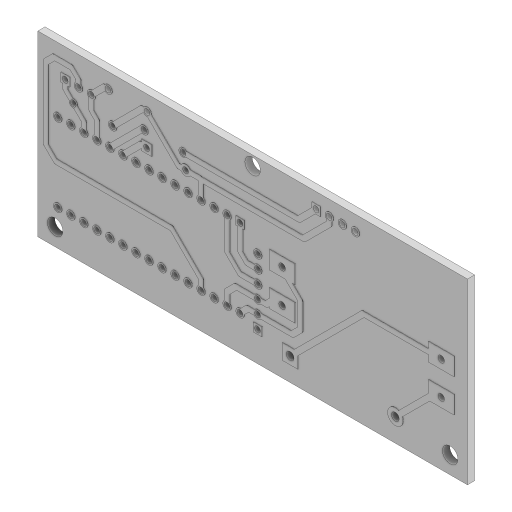
# Autodesk Inventor part: Деталь1
Saved by Autodesk Inventor 2024 (Build 280153020, 153B)
## iProperties
Created: 2023-07-24
Part Number: Деталь1
Material: Типовые
Document SubType Name: Modeling
Designer: Admin
Density: 1 g/cm^3
Appearance: По умолчанию
Author: Admin
Autodesk Inventor part; units mm, degrees
(part 1 of 3)
ref_plane "YZ Plane" through (0, 0, 0) normal (1, 0, 0) x (0, 1, 0)
ref_plane "XZ Plane" through (0, 0, 0) normal (0, 1, 0) x (-1, 0, 0)
ref_plane "XY Plane" through (0, 0, 0) normal (0, 0, 1) x (1, 0, 0)
sketch "Эскиз1" plane through (0, 0, 0) normal (0, 0, 1) x (1, 0, 0)
  line L0 (80.7425, 5.0309) -> (80.979, 4.9741)
  line L1 (80.979, 4.9741) -> (81.2037, 4.8811)
  line L2 (81.2037, 4.8811) -> (81.4111, 4.754)
  line L3 (81.4111, 4.754) -> (81.596, 4.596)
  line L4 (81.596, 4.596) -> (81.754, 4.4111)
  line L5 (81.754, 4.4111) -> (81.8811, 4.2037)
  line L6 (81.8811, 4.2037) -> (81.9741, 3.979)
  line L7 (81.9741, 3.979) -> (82.0309, 3.7425)
  line L8 (82.0309, 3.7425) -> (82.05, 3.5)
  line L9 (82.05, 3.5) -> (82.0309, 3.2575)
  line L10 (82.0309, 3.2575) -> (81.9741, 3.021)
  line L11 (81.9741, 3.021) -> (81.8811, 2.7963)
  line L12 (81.8811, 2.7963) -> (81.754, 2.5889)
  line L13 (81.754, 2.5889) -> (81.596, 2.404)
  line L14 (81.596, 2.404) -> (81.4111, 2.246)
  line L15 (81.4111, 2.246) -> (81.2037, 2.1189)
  line L16 (81.2037, 2.1189) -> (80.979, 2.0259)
  line L17 (80.979, 2.0259) -> (80.7425, 1.9691)
  line L18 (80.7425, 1.9691) -> (80.5, 1.95)
  line L19 (80.5, 1.95) -> (80.2575, 1.9691)
  line L20 (80.2575, 1.9691) -> (80.021, 2.0259)
  line L21 (80.021, 2.0259) -> (79.7963, 2.1189)
  line L22 (79.7963, 2.1189) -> (79.5889, 2.246)
  line L23 (79.5889, 2.246) -> (79.404, 2.404)
  line L24 (79.404, 2.404) -> (79.246, 2.5889)
  line L25 (79.246, 2.5889) -> (79.1189, 2.7963)
  line L26 (79.1189, 2.7963) -> (79.0259, 3.021)
  line L27 (79.0259, 3.021) -> (78.9691, 3.2575)
  line L28 (78.9691, 3.2575) -> (78.95, 3.5)
  line L29 (78.95, 3.5) -> (78.9691, 3.7425)
  line L30 (78.9691, 3.7425) -> (79.0259, 3.979)
  line L31 (79.0259, 3.979) -> (79.1189, 4.2037)
  line L32 (79.1189, 4.2037) -> (79.246, 4.4111)
  line L33 (79.246, 4.4111) -> (79.404, 4.596)
  line L34 (79.404, 4.596) -> (79.5889, 4.754)
  line L35 (79.5889, 4.754) -> (79.7963, 4.8811)
  line L36 (79.7963, 4.8811) -> (80.021, 4.9741)
  line L37 (80.021, 4.9741) -> (80.2575, 5.0309)
  line L38 (80.2575, 5.0309) -> (80.5, 5.05)
  line L39 (80.5, 5.05) -> (80.7425, 5.0309)
  line L40 (3.7425, 5.0309) -> (3.979, 4.9741)
  line L41 (3.979, 4.9741) -> (4.2037, 4.8811)
  line L42 (4.2037, 4.8811) -> (4.4111, 4.754)
  line L43 (4.4111, 4.754) -> (4.596, 4.596)
  line L44 (4.596, 4.596) -> (4.754, 4.4111)
  line L45 (4.754, 4.4111) -> (4.8811, 4.2037)
  line L46 (4.8811, 4.2037) -> (4.9741, 3.979)
  line L47 (4.9741, 3.979) -> (5.0309, 3.7425)
  line L48 (5.0309, 3.7425) -> (5.05, 3.5)
  line L49 (5.05, 3.5) -> (5.0309, 3.2575)
  line L50 (5.0309, 3.2575) -> (4.9741, 3.021)
  line L51 (4.9741, 3.021) -> (4.8811, 2.7963)
  line L52 (4.8811, 2.7963) -> (4.754, 2.5889)
  line L53 (4.754, 2.5889) -> (4.596, 2.404)
  line L54 (4.596, 2.404) -> (4.4111, 2.246)
  line L55 (4.4111, 2.246) -> (4.2037, 2.1189)
  line L56 (4.2037, 2.1189) -> (3.979, 2.0259)
  line L57 (3.979, 2.0259) -> (3.7425, 1.9691)
  line L58 (3.7425, 1.9691) -> (3.5, 1.95)
  line L59 (3.5, 1.95) -> (3.2575, 1.9691)
  line L60 (3.2575, 1.9691) -> (3.021, 2.0259)
  line L61 (3.021, 2.0259) -> (2.7963, 2.1189)
  line L62 (2.7963, 2.1189) -> (2.5889, 2.246)
  line L63 (2.5889, 2.246) -> (2.404, 2.404)
  line L64 (2.404, 2.404) -> (2.246, 2.5889)
  line L65 (2.246, 2.5889) -> (2.1189, 2.7963)
  line L66 (2.1189, 2.7963) -> (2.0259, 3.021)
  line L67 (2.0259, 3.021) -> (1.9691, 3.2575)
  line L68 (1.9691, 3.2575) -> (1.95, 3.5)
  line L69 (1.95, 3.5) -> (1.9691, 3.7425)
  line L70 (1.9691, 3.7425) -> (2.0259, 3.979)
  line L71 (2.0259, 3.979) -> (2.1189, 4.2037)
  line L72 (2.1189, 4.2037) -> (2.246, 4.4111)
  line L73 (2.246, 4.4111) -> (2.404, 4.596)
  line L74 (2.404, 4.596) -> (2.5889, 4.754)
  line L75 (2.5889, 4.754) -> (2.7963, 4.8811)
  line L76 (2.7963, 4.8811) -> (3.021, 4.9741)
  line L77 (3.021, 4.9741) -> (3.2575, 5.0309)
  line L78 (3.2575, 5.0309) -> (3.5, 5.05)
  line L79 (3.5, 5.05) -> (3.7425, 5.0309)
  line L80 (81.35, 17.15) -> (76.35, 17.15)
  line L81 (76.35, 17.15) -> (76.35, 18.4)
  line L82 (76.35, 18.4) -> (63.8171, 18.4)
  line L83 (63.8171, 18.4) -> (50.91, 5.4929)
  line L84 (50.91, 5.4929) -> (50.91, 3.2)
  line L85 (50.91, 3.2) -> (47.91, 3.2)
  line L86 (47.91, 3.2) -> (47.91, 6.2)
  line L87 (47.91, 6.2) -> (50.2029, 6.2)
  line L88 (50.2029, 6.2) -> (63.2564, 19.2536)
  line L89 (63.2564, 19.2536) -> (63.2993, 19.2856)
  line L90 (63.2993, 19.2856) -> (63.3397, 19.3206)
  line L91 (63.3397, 19.3206) -> (63.356, 19.3281)
  line L92 (63.356, 19.3281) -> (63.3704, 19.3388)
  line L93 (63.3704, 19.3388) -> (63.4205, 19.3575)
  line L94 (63.4205, 19.3575) -> (63.4691, 19.3797)
  line L95 (63.4691, 19.3797) -> (63.4869, 19.3823)
  line L96 (63.4869, 19.3823) -> (63.5037, 19.3886)
  line L97 (63.5037, 19.3886) -> (63.5571, 19.3924)
  line L98 (63.5571, 19.3924) -> (63.61, 19.4)
  line L99 (63.61, 19.4) -> (76.35, 19.4)
  line L100 (76.35, 19.4) -> (76.35, 20.65)
  line L101 (76.35, 20.65) -> (81.35, 20.65)
  line L102 (81.35, 20.65) -> (81.35, 17.15)
  line L103 (81.35, 10.7) -> (76.6071, 10.7)
  line L104 (76.6071, 10.7) -> (71.2503, 5.3431)
  line L105 (71.2503, 5.3431) -> (71.3187, 5.1871)
  line L106 (71.3187, 5.1871) -> (71.3795, 4.9469)
  line L107 (71.3795, 4.9469) -> (71.4, 4.7)
  line L108 (71.4, 4.7) -> (71.3795, 4.4531)
  line L109 (71.3795, 4.4531) -> (71.3187, 4.213)
  line L110 (71.3187, 4.213) -> (71.2192, 3.9861)
  line L111 (71.2192, 3.9861) -> (71.0837, 3.7787)
  line L112 (71.0837, 3.7787) -> (70.9159, 3.5964)
  line L113 (70.9159, 3.5964) -> (70.7204, 3.4442)
  line L114 (70.7204, 3.4442) -> (70.5025, 3.3263)
  line L115 (70.5025, 3.3263) -> (70.2682, 3.2459)
  line L116 (70.2682, 3.2459) -> (70.0239, 3.2051)
  line L117 (70.0239, 3.2051) -> (69.7761, 3.2051)
  line L118 (69.7761, 3.2051) -> (69.5318, 3.2459)
  line L119 (69.5318, 3.2459) -> (69.2975, 3.3263)
  line L120 (69.2975, 3.3263) -> (69.0796, 3.4442)
  line L121 (69.0796, 3.4442) -> (68.8841, 3.5964)
  line L122 (68.8841, 3.5964) -> (68.7163, 3.7787)
  line L123 (68.7163, 3.7787) -> (68.5808, 3.9861)
  line L124 (68.5808, 3.9861) -> (68.4813, 4.213)
  line L125 (68.4813, 4.213) -> (68.4205, 4.4531)
  line L126 (68.4205, 4.4531) -> (68.4, 4.7)
  line L127 (68.4, 4.7) -> (68.4205, 4.9469)
  line L128 (68.4205, 4.9469) -> (68.4813, 5.1871)
  line L129 (68.4813, 5.1871) -> (68.5808, 5.4139)
  line L130 (68.5808, 5.4139) -> (68.7163, 5.6213)
  line L131 (68.7163, 5.6213) -> (68.8841, 5.8036)
  line L132 (68.8841, 5.8036) -> (69.0796, 5.9558)
  line L133 (69.0796, 5.9558) -> (69.2975, 6.0737)
  line L134 (69.2975, 6.0737) -> (69.5318, 6.1541)
  line L135 (69.5318, 6.1541) -> (69.7761, 6.1949)
  line L136 (69.7761, 6.1949) -> (70.0239, 6.1949)
  line L137 (70.0239, 6.1949) -> (70.2682, 6.1541)
  line L138 (70.2682, 6.1541) -> (70.5025, 6.0737)
  line L139 (70.5025, 6.0737) -> (70.5441, 6.0512)
  line L140 (70.5441, 6.0512) -> (76.35, 11.8571)
  line L141 (76.35, 11.8571) -> (76.35, 14.2)
  line L142 (76.35, 14.2) -> (81.35, 14.2)
  line L143 (81.35, 14.2) -> (81.35, 10.7)
  line L144 (43.9, 5.16) -> (42.2, 5.16)
  line L145 (42.2, 5.16) -> (42.2, 6.86)
  line L146 (42.2, 6.86) -> (43.9, 6.86)
  line L147 (43.9, 6.86) -> (43.9, 5.16)
  line L148 (50.35, 17.2) -> (49.8571, 17.2)
  line L149 (49.8571, 17.2) -> (50.1036, 16.9536)
  line L150 (50.1036, 16.9536) -> (50.1036, 16.9535)
  line L151 (50.1036, 16.9535) -> (51.7036, 15.3536)
  line L152 (51.7036, 15.3536) -> (51.7356, 15.3107)
  line L153 (51.7356, 15.3107) -> (51.7706, 15.2703)
  line L154 (51.7706, 15.2703) -> (51.7781, 15.254)
  line L155 (51.7781, 15.254) -> (51.7888, 15.2396)
  line L156 (51.7888, 15.2396) -> (51.8075, 15.1895)
  line L157 (51.8075, 15.1895) -> (51.8297, 15.1409)
  line L158 (51.8297, 15.1409) -> (51.8323, 15.1231)
  line L159 (51.8323, 15.1231) -> (51.8386, 15.1063)
  line L160 (51.8386, 15.1063) -> (51.8424, 15.0529)
  line L161 (51.8424, 15.0529) -> (51.85, 15)
  line L162 (51.85, 15) -> (51.85, 10.1)
  line L163 (51.85, 10.1) -> (51.8424, 10.0471)
  line L164 (51.8424, 10.0471) -> (51.8386, 9.9937)
  line L165 (51.8386, 9.9937) -> (51.8323, 9.9769)
  line L166 (51.8323, 9.9769) -> (51.8297, 9.9591)
  line L167 (51.8297, 9.9591) -> (51.8075, 9.9105)
  line L168 (51.8075, 9.9105) -> (51.7888, 9.8604)
  line L169 (51.7888, 9.8604) -> (51.7781, 9.846)
  line L170 (51.7781, 9.846) -> (51.7706, 9.8297)
  line L171 (51.7706, 9.8297) -> (51.7356, 9.7893)
  line L172 (51.7356, 9.7893) -> (51.7036, 9.7464)
  line L173 (51.7036, 9.7464) -> (50.1536, 8.1965)
  line L174 (50.1536, 8.1965) -> (50.1107, 8.1644)
  line L175 (50.1107, 8.1644) -> (50.0703, 8.1294)
  line L176 (50.0703, 8.1294) -> (50.054, 8.1219)
  line L177 (50.054, 8.1219) -> (50.0396, 8.1112)
  line L178 (50.0396, 8.1112) -> (49.9895, 8.0925)
  line L179 (49.9895, 8.0925) -> (49.9409, 8.0702)
  line L180 (49.9409, 8.0702) -> (49.9231, 8.0677)
  line L181 (49.9231, 8.0677) -> (49.9063, 8.0614)
  line L182 (49.9063, 8.0614) -> (49.8529, 8.0576)
  line L183 (49.8529, 8.0576) -> (49.8, 8.05)
  line L184 (49.8, 8.05) -> (43.6743, 8.05)
  line L185 (43.6743, 8.05) -> (43.5488, 7.9245)
  line L186 (43.5488, 7.9245) -> (43.3971, 7.8292)
  line L187 (43.3971, 7.8292) -> (43.228, 7.7701)
  line L188 (43.228, 7.7701) -> (43.05, 7.75)
  line L189 (43.05, 7.75) -> (42.872, 7.7701)
  line L190 (42.872, 7.7701) -> (42.7029, 7.8292)
  line L191 (42.7029, 7.8292) -> (42.5512, 7.9245)
  line L192 (42.5512, 7.9245) -> (42.4257, 8.05)
  line L193 (42.4257, 8.05) -> (41.3167, 8.05)
  line L194 (41.3167, 8.05) -> (40.4143, 7.1476)
  line L195 (40.4143, 7.1476) -> (40.4237, 7.0641)
  line L196 (40.4237, 7.0641) -> (40.4036, 6.8861)
  line L197 (40.4036, 6.8861) -> (40.3444, 6.717)
  line L198 (40.3444, 6.717) -> (40.2491, 6.5653)
  line L199 (40.2491, 6.5653) -> (40.1225, 6.4386)
  line L200 (40.1225, 6.4386) -> (39.9708, 6.3433)
  line L201 (39.9708, 6.3433) -> (39.8017, 6.2842)
  line L202 (39.8017, 6.2842) -> (39.6237, 6.2641)
  line L203 (39.6237, 6.2641) -> (39.4456, 6.2842)
  line L204 (39.4456, 6.2842) -> (39.2766, 6.3433)
  line L205 (39.2766, 6.3433) -> (39.1249, 6.4386)
  line L206 (39.1249, 6.4386) -> (38.9982, 6.5653)
  line L207 (38.9982, 6.5653) -> (38.9029, 6.717)
  line L208 (38.9029, 6.717) -> (38.8437, 6.8861)
  line L209 (38.8437, 6.8861) -> (38.8237, 7.0641)
  line L210 (38.8237, 7.0641) -> (38.8437, 7.2421)
  line L211 (38.8437, 7.2421) -> (38.9029, 7.4112)
  line L212 (38.9029, 7.4112) -> (38.9982, 7.5629)
  line L213 (38.9982, 7.5629) -> (39.1249, 7.6896)
  line L214 (39.1249, 7.6896) -> (39.2766, 7.7849)
  line L215 (39.2766, 7.7849) -> (39.4456, 7.844)
  line L216 (39.4456, 7.844) -> (39.6237, 7.8641)
  line L217 (39.6237, 7.8641) -> (39.7071, 7.8547)
  line L218 (39.7071, 7.8547) -> (40.756, 8.9035)
  line L219 (40.756, 8.9035) -> (40.7988, 8.9356)
  line L220 (40.7988, 8.9356) -> (40.8392, 8.9706)
  line L221 (40.8392, 8.9706) -> (40.8556, 8.9781)
  line L222 (40.8556, 8.9781) -> (40.8699, 8.9888)
  line L223 (40.8699, 8.9888) -> (40.9201, 9.0075)
  line L224 (40.9201, 9.0075) -> (40.9687, 9.0297)
  line L225 (40.9687, 9.0297) -> (40.9865, 9.0323)
  line L226 (40.9865, 9.0323) -> (41.0033, 9.0386)
  line L227 (41.0033, 9.0386) -> (41.0566, 9.0424)
  line L228 (41.0566, 9.0424) -> (41.1096, 9.05)
  line L229 (41.1096, 9.05) -> (42.4257, 9.05)
  line L230 (42.4257, 9.05) -> (42.5512, 9.1755)
  line L231 (42.5512, 9.1755) -> (42.7029, 9.2708)
  line L232 (42.7029, 9.2708) -> (42.872, 9.3299)
  line L233 (42.872, 9.3299) -> (43.05, 9.35)
  line L234 (43.05, 9.35) -> (43.228, 9.3299)
  line L235 (43.228, 9.3299) -> (43.3971, 9.2708)
  line L236 (43.3971, 9.2708) -> (43.5488, 9.1755)
  line L237 (43.5488, 9.1755) -> (43.6743, 9.05)
  line L238 (43.6743, 9.05) -> (49.5929, 9.05)
  line L239 (49.5929, 9.05) -> (50.85, 10.3071)
  line L240 (50.85, 10.3071) -> (50.85, 14.7929)
  line L241 (50.85, 14.7929) -> (49.3964, 16.2464)
  line L242 (49.3964, 16.2464) -> (48.4429, 17.2)
  line L243 (48.4429, 17.2) -> (45.35, 17.2)
  line L244 (45.35, 17.2) -> (45.35, 20.7)
  line L245 (45.35, 20.7) -> (50.35, 20.7)
  line L246 (50.35, 20.7) -> (50.35, 17.2)
  line L247 (50.35, 10.7) -> (45.35, 10.7)
  line L248 (45.35, 10.7) -> (45.35, 10.9929)
  line L249 (45.35, 10.9929) -> (45.0936, 10.7364)
  line L250 (45.0936, 10.7364) -> (45.0507, 10.7044)
  line L251 (45.0507, 10.7044) -> (45.0103, 10.6694)
  line L252 (45.0103, 10.6694) -> (44.994, 10.6619)
  line L253 (44.994, 10.6619) -> (44.9796, 10.6512)
  line L254 (44.9796, 10.6512) -> (44.9295, 10.6325)
  line L255 (44.9295, 10.6325) -> (44.8809, 10.6103)
  line L256 (44.8809, 10.6103) -> (44.8631, 10.6077)
  line L257 (44.8631, 10.6077) -> (44.8463, 10.6014)
  line L258 (44.8463, 10.6014) -> (44.7929, 10.5976)
  line L259 (44.7929, 10.5976) -> (44.74, 10.59)
  line L260 (44.74, 10.59) -> (43.6743, 10.59)
  line L261 (43.6743, 10.59) -> (43.5488, 10.4645)
  line L262 (43.5488, 10.4645) -> (43.3971, 10.3692)
  line L263 (43.3971, 10.3692) -> (43.228, 10.3101)
  line L264 (43.228, 10.3101) -> (43.05, 10.29)
  line L265 (43.05, 10.29) -> (42.872, 10.3101)
  line L266 (42.872, 10.3101) -> (42.7029, 10.3692)
  line L267 (42.7029, 10.3692) -> (42.5512, 10.4645)
  line L268 (42.5512, 10.4645) -> (42.4257, 10.59)
  line L269 (42.4257, 10.59) -> (38.9971, 10.59)
  line L270 (38.9971, 10.59) -> (37.5837, 9.1766)
  line L271 (37.5837, 9.1766) -> (37.5837, 7.6884)
  line L272 (37.5837, 7.6884) -> (37.7091, 7.5629)
  line L273 (37.7091, 7.5629) -> (37.8044, 7.4112)
  line L274 (37.8044, 7.4112) -> (37.8636, 7.2421)
  line L275 (37.8636, 7.2421) -> (37.8837, 7.0641)
  line L276 (37.8837, 7.0641) -> (37.8636, 6.8861)
  line L277 (37.8636, 6.8861) -> (37.8044, 6.717)
  line L278 (37.8044, 6.717) -> (37.7091, 6.5653)
  line L279 (37.7091, 6.5653) -> (37.5825, 6.4386)
  line L280 (37.5825, 6.4386) -> (37.4308, 6.3433)
  line L281 (37.4308, 6.3433) -> (37.2617, 6.2842)
  line L282 (37.2617, 6.2842) -> (37.0837, 6.2641)
  line L283 (37.0837, 6.2641) -> (36.9056, 6.2842)
  line L284 (36.9056, 6.2842) -> (36.7366, 6.3433)
  line L285 (36.7366, 6.3433) -> (36.5849, 6.4386)
  line L286 (36.5849, 6.4386) -> (36.4582, 6.5653)
  line L287 (36.4582, 6.5653) -> (36.3629, 6.717)
  line L288 (36.3629, 6.717) -> (36.3037, 6.8861)
  line L289 (36.3037, 6.8861) -> (36.2837, 7.0641)
  line L290 (36.2837, 7.0641) -> (36.3037, 7.2421)
  line L291 (36.3037, 7.2421) -> (36.3629, 7.4112)
  line L292 (36.3629, 7.4112) -> (36.4582, 7.5629)
  line L293 (36.4582, 7.5629) -> (36.5837, 7.6884)
  line L294 (36.5837, 7.6884) -> (36.5837, 9.3837)
  line L295 (36.5837, 9.3837) -> (36.5913, 9.4366)
  line L296 (36.5913, 9.4366) -> (36.5951, 9.4899)
  line L297 (36.5951, 9.4899) -> (36.6014, 9.5068)
  line L298 (36.6014, 9.5068) -> (36.6039, 9.5245)
  line L299 (36.6039, 9.5245) -> (36.6261, 9.5732)
  line L300 (36.6261, 9.5732) -> (36.6448, 9.6233)
  line L301 (36.6448, 9.6233) -> (36.6556, 9.6377)
  line L302 (36.6556, 9.6377) -> (36.663, 9.654)
  line L303 (36.663, 9.654) -> (36.6981, 9.6944)
  line L304 (36.6981, 9.6944) -> (36.7301, 9.7372)
  line L305 (36.7301, 9.7372) -> (38.4364, 11.4436)
  line L306 (38.4364, 11.4436) -> (38.4793, 11.4756)
  line L307 (38.4793, 11.4756) -> (38.5197, 11.5106)
  line L308 (38.5197, 11.5106) -> (38.536, 11.5181)
  line L309 (38.536, 11.5181) -> (38.5504, 11.5288)
  line L310 (38.5504, 11.5288) -> (38.6005, 11.5475)
  line L311 (38.6005, 11.5475) -> (38.6491, 11.5697)
  line L312 (38.6491, 11.5697) -> (38.6669, 11.5723)
  line L313 (38.6669, 11.5723) -> (38.6837, 11.5786)
  line L314 (38.6837, 11.5786) -> (38.7371, 11.5824)
  line L315 (38.7371, 11.5824) -> (38.79, 11.59)
  line L316 (38.79, 11.59) -> (42.4257, 11.59)
  line L317 (42.4257, 11.59) -> (42.5512, 11.7155)
  line L318 (42.5512, 11.7155) -> (42.7029, 11.8108)
  line L319 (42.7029, 11.8108) -> (42.872, 11.8699)
  line L320 (42.872, 11.8699) -> (43.05, 11.89)
  line L321 (43.05, 11.89) -> (43.228, 11.8699)
  line L322 (43.228, 11.8699) -> (43.3971, 11.8108)
  line L323 (43.3971, 11.8108) -> (43.5488, 11.7155)
  line L324 (43.5488, 11.7155) -> (43.6743, 11.59)
  line L325 (43.6743, 11.59) -> (44.5329, 11.59)
  line L326 (44.5329, 11.59) -> (45.35, 12.4071)
  line L327 (45.35, 12.4071) -> (45.35, 14.2)
  line L328 (45.35, 14.2) -> (50.35, 14.2)
  line L329 (50.35, 14.2) -> (50.35, 10.7)
  line L330 (34.7217, 7.844) -> (34.8908, 7.7849)
  line L331 (34.8908, 7.7849) -> (35.0425, 7.6896)
  line L332 (35.0425, 7.6896) -> (35.1691, 7.5629)
  line L333 (35.1691, 7.5629) -> (35.2644, 7.4112)
  line L334 (35.2644, 7.4112) -> (35.3236, 7.2421)
  line L335 (35.3236, 7.2421) -> (35.3437, 7.0641)
  line L336 (35.3437, 7.0641) -> (35.3236, 6.8861)
  line L337 (35.3236, 6.8861) -> (35.2644, 6.717)
  line L338 (35.2644, 6.717) -> (35.1691, 6.5653)
  line L339 (35.1691, 6.5653) -> (35.0425, 6.4386)
  line L340 (35.0425, 6.4386) -> (34.8908, 6.3433)
  line L341 (34.8908, 6.3433) -> (34.7217, 6.2842)
  line L342 (34.7217, 6.2842) -> (34.5437, 6.2641)
  line L343 (34.5437, 6.2641) -> (34.3656, 6.2842)
  line L344 (34.3656, 6.2842) -> (34.1966, 6.3433)
  line L345 (34.1966, 6.3433) -> (34.0449, 6.4386)
  line L346 (34.0449, 6.4386) -> (33.9182, 6.5653)
  line L347 (33.9182, 6.5653) -> (33.8229, 6.717)
  line L348 (33.8229, 6.717) -> (33.7637, 6.8861)
  line L349 (33.7637, 6.8861) -> (33.7437, 7.0641)
  line L350 (33.7437, 7.0641) -> (33.7637, 7.2421)
  line L351 (33.7637, 7.2421) -> (33.8229, 7.4112)
  line L352 (33.8229, 7.4112) -> (33.9182, 7.5629)
  line L353 (33.9182, 7.5629) -> (34.0449, 7.6896)
  line L354 (34.0449, 7.6896) -> (34.1966, 7.7849)
  line L355 (34.1966, 7.7849) -> (34.3656, 7.844)
  line L356 (34.3656, 7.844) -> (34.5437, 7.8641)
  line L357 (34.5437, 7.8641) -> (34.7217, 7.844)
  line L358 (6.7836, 32.5755) -> (6.8369, 32.5717)
  line L359 (6.8369, 32.5717) -> (6.8538, 32.5654)
  line L360 (6.8538, 32.5654) -> (6.8715, 32.5628)
  line L361 (6.8715, 32.5628) -> (6.9202, 32.5406)
  line L362 (6.9202, 32.5406) -> (6.9703, 32.5219)
  line L363 (6.9703, 32.5219) -> (6.9847, 32.5112)
  line L364 (6.9847, 32.5112) -> (7.001, 32.5037)
  line L365 (7.001, 32.5037) -> (7.0414, 32.4687)
  line L366 (7.0414, 32.4687) -> (7.0842, 32.4366)
  line L367 (7.0842, 32.4366) -> (8.4545, 31.0663)
  line L368 (8.4545, 31.0663) -> (8.4866, 31.0235)
  line L369 (8.4866, 31.0235) -> (8.5216, 30.9831)
  line L370 (8.5216, 30.9831) -> (8.529, 30.9668)
  line L371 (8.529, 30.9668) -> (8.5398, 30.9524)
  line L372 (8.5398, 30.9524) -> (8.5585, 30.9023)
  line L373 (8.5585, 30.9023) -> (8.5807, 30.8537)
  line L374 (8.5807, 30.8537) -> (8.5833, 30.8359)
  line L375 (8.5833, 30.8359) -> (8.5895, 30.8191)
  line L376 (8.5895, 30.8191) -> (8.5933, 30.7657)
  line L377 (8.5933, 30.7657) -> (8.601, 30.7128)
  line L378 (8.601, 30.7128) -> (8.601, 30.0483)
  line L379 (8.601, 30.0483) -> (8.7264, 29.9229)
  line L380 (8.7264, 29.9229) -> (8.8217, 29.7712)
  line L381 (8.8217, 29.7712) -> (8.8809, 29.6021)
  line L382 (8.8809, 29.6021) -> (8.901, 29.4241)
  line L383 (8.901, 29.4241) -> (8.8809, 29.2461)
  line L384 (8.8809, 29.2461) -> (8.8217, 29.077)
  line L385 (8.8217, 29.077) -> (8.7264, 28.9253)
  line L386 (8.7264, 28.9253) -> (8.5998, 28.7986)
  line L387 (8.5998, 28.7986) -> (8.4481, 28.7033)
  line L388 (8.4481, 28.7033) -> (8.279, 28.6441)
  line L389 (8.279, 28.6441) -> (8.101, 28.6241)
  line L390 (8.101, 28.6241) -> (7.9229, 28.6441)
  line L391 (7.9229, 28.6441) -> (7.7538, 28.7033)
  line L392 (7.7538, 28.7033) -> (7.6022, 28.7986)
  line L393 (7.6022, 28.7986) -> (7.4755, 28.9253)
  line L394 (7.4755, 28.9253) -> (7.3802, 29.077)
  line L395 (7.3802, 29.077) -> (7.321, 29.2461)
  line L396 (7.321, 29.2461) -> (7.301, 29.4241)
  line L397 (7.301, 29.4241) -> (7.321, 29.6021)
  line L398 (7.321, 29.6021) -> (7.3802, 29.7712)
  line L399 (7.3802, 29.7712) -> (7.4755, 29.9229)
  line L400 (7.4755, 29.9229) -> (7.601, 30.0483)
  line L401 (7.601, 30.0483) -> (7.601, 30.5057)
  line L402 (7.601, 30.5057) -> (6.5236, 31.5831)
  line L403 (6.5236, 31.5831) -> (3.5088, 31.5831)
  line L404 (3.5088, 31.5831) -> (2.2777, 30.352)
  line L405 (2.2777, 30.352) -> (2.2777, 16.7962)
  line L406 (2.2777, 16.7962) -> (3.8898, 15.1841)
  line L407 (3.8898, 15.1841) -> (26.2887, 15.1841)
  line L408 (26.2887, 15.1841) -> (26.3416, 15.1765)
  line L409 (26.3416, 15.1765) -> (26.3949, 15.1727)
  line L410 (26.3949, 15.1727) -> (26.4118, 15.1664)
  line L411 (26.4118, 15.1664) -> (26.4295, 15.1638)
  line L412 (26.4295, 15.1638) -> (26.4782, 15.1416)
  line L413 (26.4782, 15.1416) -> (26.5283, 15.1229)
  line L414 (26.5283, 15.1229) -> (26.5426, 15.1122)
  line L415 (26.5426, 15.1122) -> (26.559, 15.1047)
  line L416 (26.559, 15.1047) -> (26.5994, 15.0697)
  line L417 (26.5994, 15.0697) -> (26.6422, 15.0376)
  line L418 (26.6422, 15.0376) -> (32.3572, 9.3226)
  line L419 (32.3572, 9.3226) -> (32.3893, 9.2798)
  line L420 (32.3893, 9.2798) -> (32.4243, 9.2394)
  line L421 (32.4243, 9.2394) -> (32.4317, 9.2231)
  line L422 (32.4317, 9.2231) -> (32.4425, 9.2087)
  line L423 (32.4425, 9.2087) -> (32.4612, 9.1586)
  line L424 (32.4612, 9.1586) -> (32.4834, 9.11)
  line L425 (32.4834, 9.11) -> (32.486, 9.0922)
  line L426 (32.486, 9.0922) -> (32.4922, 9.0754)
  line L427 (32.4922, 9.0754) -> (32.496, 9.022)
  line L428 (32.496, 9.022) -> (32.5037, 8.9691)
  line L429 (32.5037, 8.9691) -> (32.5037, 7.6884)
  line L430 (32.5037, 7.6884) -> (32.6291, 7.5629)
  line L431 (32.6291, 7.5629) -> (32.7244, 7.4112)
  line L432 (32.7244, 7.4112) -> (32.7836, 7.2421)
  line L433 (32.7836, 7.2421) -> (32.8037, 7.0641)
  line L434 (32.8037, 7.0641) -> (32.7836, 6.8861)
  line L435 (32.7836, 6.8861) -> (32.7244, 6.717)
  line L436 (32.7244, 6.717) -> (32.6291, 6.5653)
  line L437 (32.6291, 6.5653) -> (32.5025, 6.4386)
  line L438 (32.5025, 6.4386) -> (32.3508, 6.3433)
  line L439 (32.3508, 6.3433) -> (32.1817, 6.2842)
  line L440 (32.1817, 6.2842) -> (32.0037, 6.2641)
  line L441 (32.0037, 6.2641) -> (31.8256, 6.2842)
  line L442 (31.8256, 6.2842) -> (31.6566, 6.3433)
  line L443 (31.6566, 6.3433) -> (31.5049, 6.4386)
  line L444 (31.5049, 6.4386) -> (31.3782, 6.5653)
  line L445 (31.3782, 6.5653) -> (31.2829, 6.717)
  line L446 (31.2829, 6.717) -> (31.2237, 6.8861)
  line L447 (31.2237, 6.8861) -> (31.2037, 7.0641)
  line L448 (31.2037, 7.0641) -> (31.2237, 7.2421)
  line L449 (31.2237, 7.2421) -> (31.2829, 7.4112)
  line L450 (31.2829, 7.4112) -> (31.3782, 7.5629)
  line L451 (31.3782, 7.5629) -> (31.5037, 7.6884)
  line L452 (31.5037, 7.6884) -> (31.5037, 8.762)
  line L453 (31.5037, 8.762) -> (26.0816, 14.1841)
  line L454 (26.0816, 14.1841) -> (3.6827, 14.1841)
  line L455 (3.6827, 14.1841) -> (3.6297, 14.1917)
  line L456 (3.6297, 14.1917) -> (3.5764, 14.1955)
  line L457 (3.5764, 14.1955) -> (3.5596, 14.2018)
  line L458 (3.5596, 14.2018) -> (3.5418, 14.2043)
  line L459 (3.5418, 14.2043) -> (3.4931, 14.2266)
  line L460 (3.4931, 14.2266) -> (3.443, 14.2453)
  line L461 (3.443, 14.2453) -> (3.4287, 14.256)
  line L462 (3.4287, 14.256) -> (3.4123, 14.2635)
  line L463 (3.4123, 14.2635) -> (3.3719, 14.2985)
  line L464 (3.3719, 14.2985) -> (3.3291, 14.3305)
  line L465 (3.3291, 14.3305) -> (1.4241, 16.2355)
  line L466 (1.4241, 16.2355) -> (1.3921, 16.2783)
  line L467 (1.3921, 16.2783) -> (1.357, 16.3188)
  line L468 (1.357, 16.3188) -> (1.3496, 16.3351)
  line L469 (1.3496, 16.3351) -> (1.3388, 16.3495)
  line L470 (1.3388, 16.3495) -> (1.3201, 16.3996)
  line L471 (1.3201, 16.3996) -> (1.2979, 16.4482)
  line L472 (1.2979, 16.4482) -> (1.2954, 16.466)
  line L473 (1.2954, 16.466) -> (1.2891, 16.4828)
  line L474 (1.2891, 16.4828) -> (1.2853, 16.5362)
  line L475 (1.2853, 16.5362) -> (1.2777, 16.5891)
  line L476 (1.2777, 16.5891) -> (1.2777, 30.5591)
  line L477 (1.2777, 30.5591) -> (1.2853, 30.612)
  line L478 (1.2853, 30.612) -> (1.2891, 30.6654)
  line L479 (1.2891, 30.6654) -> (1.2954, 30.6822)
  line L480 (1.2954, 30.6822) -> (1.2979, 30.7)
  line L481 (1.2979, 30.7) -> (1.3201, 30.7486)
  line L482 (1.3201, 30.7486) -> (1.3388, 30.7987)
  line L483 (1.3388, 30.7987) -> (1.3496, 30.8131)
  line L484 (1.3496, 30.8131) -> (1.357, 30.8294)
  line L485 (1.357, 30.8294) -> (1.3921, 30.8698)
  line L486 (1.3921, 30.8698) -> (1.4241, 30.9126)
  line L487 (1.4241, 30.9126) -> (2.9481, 32.4366)
  line L488 (2.9481, 32.4366) -> (2.9909, 32.4687)
  line L489 (2.9909, 32.4687) -> (3.0313, 32.5037)
  line L490 (3.0313, 32.5037) -> (3.0477, 32.5112)
  line L491 (3.0477, 32.5112) -> (3.062, 32.5219)
  line L492 (3.062, 32.5219) -> (3.1121, 32.5406)
  line L493 (3.1121, 32.5406) -> (3.1608, 32.5628)
  line L494 (3.1608, 32.5628) -> (3.1786, 32.5654)
  line L495 (3.1786, 32.5654) -> (3.1954, 32.5717)
  line L496 (3.1954, 32.5717) -> (3.2487, 32.5755)
  line L497 (3.2487, 32.5755) -> (3.3017, 32.5831)
  line L498 (3.3017, 32.5831) -> (6.7307, 32.5831)
  line L499 (6.7307, 32.5831) -> (6.7836, 32.5755)
  line L500 (29.6417, 7.844) -> (29.8108, 7.7849)
  line L501 (29.8108, 7.7849) -> (29.9625, 7.6896)
  line L502 (29.9625, 7.6896) -> (30.0891, 7.5629)
  line L503 (30.0891, 7.5629) -> (30.1844, 7.4112)
  line L504 (30.1844, 7.4112) -> (30.2436, 7.2421)
  line L505 (30.2436, 7.2421) -> (30.2637, 7.0641)
  line L506 (30.2637, 7.0641) -> (30.2436, 6.8861)
  line L507 (30.2436, 6.8861) -> (30.1844, 6.717)
  line L508 (30.1844, 6.717) -> (30.0891, 6.5653)
  line L509 (30.0891, 6.5653) -> (29.9625, 6.4386)
  line L510 (29.9625, 6.4386) -> (29.8108, 6.3433)
  line L511 (29.8108, 6.3433) -> (29.6417, 6.2842)
  line L512 (29.6417, 6.2842) -> (29.4637, 6.2641)
  line L513 (29.4637, 6.2641) -> (29.2856, 6.2842)
  line L514 (29.2856, 6.2842) -> (29.1166, 6.3433)
  line L515 (29.1166, 6.3433) -> (28.9649, 6.4386)
  line L516 (28.9649, 6.4386) -> (28.8382, 6.5653)
  line L517 (28.8382, 6.5653) -> (28.7429, 6.717)
  line L518 (28.7429, 6.717) -> (28.6837, 6.8861)
  line L519 (28.6837, 6.8861) -> (28.6637, 7.0641)
  line L520 (28.6637, 7.0641) -> (28.6837, 7.2421)
  line L521 (28.6837, 7.2421) -> (28.7429, 7.4112)
  line L522 (28.7429, 7.4112) -> (28.8382, 7.5629)
  line L523 (28.8382, 7.5629) -> (28.9649, 7.6896)
  line L524 (28.9649, 7.6896) -> (29.1166, 7.7849)
  line L525 (29.1166, 7.7849) -> (29.2856, 7.844)
  line L526 (29.2856, 7.844) -> (29.4637, 7.8641)
  line L527 (29.4637, 7.8641) -> (29.6417, 7.844)
  line L528 (27.1017, 7.844) -> (27.2708, 7.7849)
  line L529 (27.2708, 7.7849) -> (27.4225, 7.6896)
  line L530 (27.4225, 7.6896) -> (27.5491, 7.5629)
  line L531 (27.5491, 7.5629) -> (27.6444, 7.4112)
  line L532 (27.6444, 7.4112) -> (27.7036, 7.2421)
  line L533 (27.7036, 7.2421) -> (27.7237, 7.0641)
  line L534 (27.7237, 7.0641) -> (27.7036, 6.8861)
  line L535 (27.7036, 6.8861) -> (27.6444, 6.717)
  line L536 (27.6444, 6.717) -> (27.5491, 6.5653)
  line L537 (27.5491, 6.5653) -> (27.4225, 6.4386)
  line L538 (27.4225, 6.4386) -> (27.2708, 6.3433)
  line L539 (27.2708, 6.3433) -> (27.1017, 6.2842)
  line L540 (27.1017, 6.2842) -> (26.9237, 6.2641)
  line L541 (26.9237, 6.2641) -> (26.7456, 6.2842)
  line L542 (26.7456, 6.2842) -> (26.5766, 6.3433)
  line L543 (26.5766, 6.3433) -> (26.4249, 6.4386)
  line L544 (26.4249, 6.4386) -> (26.2982, 6.5653)
  line L545 (26.2982, 6.5653) -> (26.2029, 6.717)
  line L546 (26.2029, 6.717) -> (26.1437, 6.8861)
  line L547 (26.1437, 6.8861) -> (26.1237, 7.0641)
  line L548 (26.1237, 7.0641) -> (26.1437, 7.2421)
  line L549 (26.1437, 7.2421) -> (26.2029, 7.4112)
  line L550 (26.2029, 7.4112) -> (26.2982, 7.5629)
  line L551 (26.2982, 7.5629) -> (26.4249, 7.6896)
  line L552 (26.4249, 7.6896) -> (26.5766, 7.7849)
  line L553 (26.5766, 7.7849) -> (26.7456, 7.844)
  line L554 (26.7456, 7.844) -> (26.9237, 7.8641)
  line L555 (26.9237, 7.8641) -> (27.1017, 7.844)
  line L556 (24.5617, 7.844) -> (24.7308, 7.7849)
  line L557 (24.7308, 7.7849) -> (24.8825, 7.6896)
  line L558 (24.8825, 7.6896) -> (25.0091, 7.5629)
  line L559 (25.0091, 7.5629) -> (25.1044, 7.4112)
  line L560 (25.1044, 7.4112) -> (25.1636, 7.2421)
  line L561 (25.1636, 7.2421) -> (25.1837, 7.0641)
  line L562 (25.1837, 7.0641) -> (25.1636, 6.8861)
  line L563 (25.1636, 6.8861) -> (25.1044, 6.717)
  line L564 (25.1044, 6.717) -> (25.0091, 6.5653)
  line L565 (25.0091, 6.5653) -> (24.8825, 6.4386)
  line L566 (24.8825, 6.4386) -> (24.7308, 6.3433)
  line L567 (24.7308, 6.3433) -> (24.5617, 6.2842)
  line L568 (24.5617, 6.2842) -> (24.3837, 6.2641)
  line L569 (24.3837, 6.2641) -> (24.2056, 6.2842)
  line L570 (24.2056, 6.2842) -> (24.0366, 6.3433)
  line L571 (24.0366, 6.3433) -> (23.8849, 6.4386)
  line L572 (23.8849, 6.4386) -> (23.7582, 6.5653)
  line L573 (23.7582, 6.5653) -> (23.6629, 6.717)
  line L574 (23.6629, 6.717) -> (23.6037, 6.8861)
  line L575 (23.6037, 6.8861) -> (23.5837, 7.0641)
  line L576 (23.5837, 7.0641) -> (23.6037, 7.2421)
  line L577 (23.6037, 7.2421) -> (23.6629, 7.4112)
  line L578 (23.6629, 7.4112) -> (23.7582, 7.5629)
  line L579 (23.7582, 7.5629) -> (23.8849, 7.6896)
  line L580 (23.8849, 7.6896) -> (24.0366, 7.7849)
  line L581 (24.0366, 7.7849) -> (24.2056, 7.844)
  line L582 (24.2056, 7.844) -> (24.3837, 7.8641)
  line L583 (24.3837, 7.8641) -> (24.5617, 7.844)
  line L584 (22.0217, 7.844) -> (22.1908, 7.7849)
  line L585 (22.1908, 7.7849) -> (22.3425, 7.6896)
  line L586 (22.3425, 7.6896) -> (22.4691, 7.5629)
  line L587 (22.4691, 7.5629) -> (22.5644, 7.4112)
  line L588 (22.5644, 7.4112) -> (22.6236, 7.2421)
  line L589 (22.6236, 7.2421) -> (22.6437, 7.0641)
  line L590 (22.6437, 7.0641) -> (22.6236, 6.8861)
  line L591 (22.6236, 6.8861) -> (22.5644, 6.717)
  line L592 (22.5644, 6.717) -> (22.4691, 6.5653)
  line L593 (22.4691, 6.5653) -> (22.3425, 6.4386)
  line L594 (22.3425, 6.4386) -> (22.1908, 6.3433)
  line L595 (22.1908, 6.3433) -> (22.0217, 6.2842)
  line L596 (22.0217, 6.2842) -> (21.8437, 6.2641)
  line L597 (21.8437, 6.2641) -> (21.6656, 6.2842)
  line L598 (21.6656, 6.2842) -> (21.4966, 6.3433)
  line L599 (21.4966, 6.3433) -> (21.3449, 6.4386)
  line L600 (21.3449, 6.4386) -> (21.2182, 6.5653)
  line L601 (21.2182, 6.5653) -> (21.1229, 6.717)
  line L602 (21.1229, 6.717) -> (21.0637, 6.8861)
  line L603 (21.0637, 6.8861) -> (21.0437, 7.0641)
  line L604 (21.0437, 7.0641) -> (21.0637, 7.2421)
  line L605 (21.0637, 7.2421) -> (21.1229, 7.4112)
  line L606 (21.1229, 7.4112) -> (21.2182, 7.5629)
  line L607 (21.2182, 7.5629) -> (21.3449, 7.6896)
  line L608 (21.3449, 7.6896) -> (21.4966, 7.7849)
  line L609 (21.4966, 7.7849) -> (21.6656, 7.844)
  line L610 (21.6656, 7.844) -> (21.8437, 7.8641)
  line L611 (21.8437, 7.8641) -> (22.0217, 7.844)
  line L612 (19.4817, 7.844) -> (19.6508, 7.7849)
  line L613 (19.6508, 7.7849) -> (19.8025, 7.6896)
  line L614 (19.8025, 7.6896) -> (19.9291, 7.5629)
  line L615 (19.9291, 7.5629) -> (20.0244, 7.4112)
  line L616 (20.0244, 7.4112) -> (20.0836, 7.2421)
  line L617 (20.0836, 7.2421) -> (20.1037, 7.0641)
  line L618 (20.1037, 7.0641) -> (20.0836, 6.8861)
  line L619 (20.0836, 6.8861) -> (20.0244, 6.717)
  line L620 (20.0244, 6.717) -> (19.9291, 6.5653)
  line L621 (19.9291, 6.5653) -> (19.8025, 6.4386)
  line L622 (19.8025, 6.4386) -> (19.6508, 6.3433)
  line L623 (19.6508, 6.3433) -> (19.4817, 6.2842)
  line L624 (19.4817, 6.2842) -> (19.3037, 6.2641)
  line L625 (19.3037, 6.2641) -> (19.1256, 6.2842)
  line L626 (19.1256, 6.2842) -> (18.9566, 6.3433)
  line L627 (18.9566, 6.3433) -> (18.8049, 6.4386)
  line L628 (18.8049, 6.4386) -> (18.6782, 6.5653)
  line L629 (18.6782, 6.5653) -> (18.5829, 6.717)
  line L630 (18.5829, 6.717) -> (18.5237, 6.8861)
  line L631 (18.5237, 6.8861) -> (18.5037, 7.0641)
  line L632 (18.5037, 7.0641) -> (18.5237, 7.2421)
  line L633 (18.5237, 7.2421) -> (18.5829, 7.4112)
  line L634 (18.5829, 7.4112) -> (18.6782, 7.5629)
  line L635 (18.6782, 7.5629) -> (18.8049, 7.6896)
  line L636 (18.8049, 7.6896) -> (18.9566, 7.7849)
  line L637 (18.9566, 7.7849) -> (19.1256, 7.844)
  line L638 (19.1256, 7.844) -> (19.3037, 7.8641)
  line L639 (19.3037, 7.8641) -> (19.4817, 7.844)
  line L640 (16.9417, 7.844) -> (17.1108, 7.7849)
  line L641 (17.1108, 7.7849) -> (17.2625, 7.6896)
  line L642 (17.2625, 7.6896) -> (17.3891, 7.5629)
  line L643 (17.3891, 7.5629) -> (17.4844, 7.4112)
  line L644 (17.4844, 7.4112) -> (17.5436, 7.2421)
  line L645 (17.5436, 7.2421) -> (17.5637, 7.0641)
  line L646 (17.5637, 7.0641) -> (17.5436, 6.8861)
  line L647 (17.5436, 6.8861) -> (17.4844, 6.717)
  line L648 (17.4844, 6.717) -> (17.3891, 6.5653)
  line L649 (17.3891, 6.5653) -> (17.2625, 6.4386)
  line L650 (17.2625, 6.4386) -> (17.1108, 6.3433)
  line L651 (17.1108, 6.3433) -> (16.9417, 6.2842)
  line L652 (16.9417, 6.2842) -> (16.7637, 6.2641)
  line L653 (16.7637, 6.2641) -> (16.5856, 6.2842)
  line L654 (16.5856, 6.2842) -> (16.4166, 6.3433)
  line L655 (16.4166, 6.3433) -> (16.2649, 6.4386)
  line L656 (16.2649, 6.4386) -> (16.1382, 6.5653)
  line L657 (16.1382, 6.5653) -> (16.0429, 6.717)
  line L658 (16.0429, 6.717) -> (15.9837, 6.8861)
  line L659 (15.9837, 6.8861) -> (15.9637, 7.0641)
  line L660 (15.9637, 7.0641) -> (15.9837, 7.2421)
  line L661 (15.9837, 7.2421) -> (16.0429, 7.4112)
  line L662 (16.0429, 7.4112) -> (16.1382, 7.5629)
  line L663 (16.1382, 7.5629) -> (16.2649, 7.6896)
  line L664 (16.2649, 7.6896) -> (16.4166, 7.7849)
  line L665 (16.4166, 7.7849) -> (16.5856, 7.844)
  line L666 (16.5856, 7.844) -> (16.7637, 7.8641)
  line L667 (16.7637, 7.8641) -> (16.9417, 7.844)
  line L668 (14.4017, 7.844) -> (14.5708, 7.7849)
  line L669 (14.5708, 7.7849) -> (14.7225, 7.6896)
  line L670 (14.7225, 7.6896) -> (14.8491, 7.5629)
  line L671 (14.8491, 7.5629) -> (14.9444, 7.4112)
  line L672 (14.9444, 7.4112) -> (15.0036, 7.2421)
  line L673 (15.0036, 7.2421) -> (15.0237, 7.0641)
  line L674 (15.0237, 7.0641) -> (15.0036, 6.8861)
  line L675 (15.0036, 6.8861) -> (14.9444, 6.717)
  line L676 (14.9444, 6.717) -> (14.8491, 6.5653)
  line L677 (14.8491, 6.5653) -> (14.7225, 6.4386)
  line L678 (14.7225, 6.4386) -> (14.5708, 6.3433)
  line L679 (14.5708, 6.3433) -> (14.4017, 6.2842)
  line L680 (14.4017, 6.2842) -> (14.2237, 6.2641)
  line L681 (14.2237, 6.2641) -> (14.0456, 6.2842)
  line L682 (14.0456, 6.2842) -> (13.8766, 6.3433)
  line L683 (13.8766, 6.3433) -> (13.7249, 6.4386)
  line L684 (13.7249, 6.4386) -> (13.5982, 6.5653)
  line L685 (13.5982, 6.5653) -> (13.5029, 6.717)
  line L686 (13.5029, 6.717) -> (13.4437, 6.8861)
  line L687 (13.4437, 6.8861) -> (13.4237, 7.0641)
  line L688 (13.4237, 7.0641) -> (13.4437, 7.2421)
  line L689 (13.4437, 7.2421) -> (13.5029, 7.4112)
  line L690 (13.5029, 7.4112) -> (13.5982, 7.5629)
  line L691 (13.5982, 7.5629) -> (13.7249, 7.6896)
  line L692 (13.7249, 7.6896) -> (13.8766, 7.7849)
  line L693 (13.8766, 7.7849) -> (14.0456, 7.844)
  line L694 (14.0456, 7.844) -> (14.2237, 7.8641)
  line L695 (14.2237, 7.8641) -> (14.4017, 7.844)
  line L696 (11.8617, 7.844) -> (12.0308, 7.7849)
  line L697 (12.0308, 7.7849) -> (12.1825, 7.6896)
  line L698 (12.1825, 7.6896) -> (12.3091, 7.5629)
  line L699 (12.3091, 7.5629) -> (12.4044, 7.4112)
  line L700 (12.4044, 7.4112) -> (12.4636, 7.2421)
  line L701 (12.4636, 7.2421) -> (12.4837, 7.0641)
  line L702 (12.4837, 7.0641) -> (12.4636, 6.8861)
  line L703 (12.4636, 6.8861) -> (12.4044, 6.717)
  line L704 (12.4044, 6.717) -> (12.3091, 6.5653)
  line L705 (12.3091, 6.5653) -> (12.1825, 6.4386)
  line L706 (12.1825, 6.4386) -> (12.0308, 6.3433)
  line L707 (12.0308, 6.3433) -> (11.8617, 6.2842)
  line L708 (11.8617, 6.2842) -> (11.6837, 6.2641)
  line L709 (11.6837, 6.2641) -> (11.5056, 6.2842)
  line L710 (11.5056, 6.2842) -> (11.3366, 6.3433)
  line L711 (11.3366, 6.3433) -> (11.1849, 6.4386)
  line L712 (11.1849, 6.4386) -> (11.0582, 6.5653)
  line L713 (11.0582, 6.5653) -> (10.9629, 6.717)
  line L714 (10.9629, 6.717) -> (10.9037, 6.8861)
  line L715 (10.9037, 6.8861) -> (10.8837, 7.0641)
  line L716 (10.8837, 7.0641) -> (10.9037, 7.2421)
  line L717 (10.9037, 7.2421) -> (10.9629, 7.4112)
  line L718 (10.9629, 7.4112) -> (11.0582, 7.5629)
  line L719 (11.0582, 7.5629) -> (11.1849, 7.6896)
  line L720 (11.1849, 7.6896) -> (11.3366, 7.7849)
  line L721 (11.3366, 7.7849) -> (11.5056, 7.844)
  line L722 (11.5056, 7.844) -> (11.6837, 7.8641)
  line L723 (11.6837, 7.8641) -> (11.8617, 7.844)
  line L724 (9.3217, 7.844) -> (9.4908, 7.7849)
  line L725 (9.4908, 7.7849) -> (9.6425, 7.6896)
  line L726 (9.6425, 7.6896) -> (9.7691, 7.5629)
  line L727 (9.7691, 7.5629) -> (9.8644, 7.4112)
  line L728 (9.8644, 7.4112) -> (9.9236, 7.2421)
  line L729 (9.9236, 7.2421) -> (9.9437, 7.0641)
  line L730 (9.9437, 7.0641) -> (9.9236, 6.8861)
  line L731 (9.9236, 6.8861) -> (9.8644, 6.717)
  line L732 (9.8644, 6.717) -> (9.7691, 6.5653)
  line L733 (9.7691, 6.5653) -> (9.6425, 6.4386)
  line L734 (9.6425, 6.4386) -> (9.4908, 6.3433)
  line L735 (9.4908, 6.3433) -> (9.3217, 6.2842)
  line L736 (9.3217, 6.2842) -> (9.1437, 6.2641)
  line L737 (9.1437, 6.2641) -> (8.9656, 6.2842)
  line L738 (8.9656, 6.2842) -> (8.7965, 6.3433)
  line L739 (8.7965, 6.3433) -> (8.6449, 6.4386)
  line L740 (8.6449, 6.4386) -> (8.5182, 6.5653)
  line L741 (8.5182, 6.5653) -> (8.4229, 6.717)
  line L742 (8.4229, 6.717) -> (8.3637, 6.8861)
  line L743 (8.3637, 6.8861) -> (8.3437, 7.0641)
  line L744 (8.3437, 7.0641) -> (8.3637, 7.2421)
  line L745 (8.3637, 7.2421) -> (8.4229, 7.4112)
  line L746 (8.4229, 7.4112) -> (8.5182, 7.5629)
  line L747 (8.5182, 7.5629) -> (8.6449, 7.6896)
  line L748 (8.6449, 7.6896) -> (8.7965, 7.7849)
  line L749 (8.7965, 7.7849) -> (8.9656, 7.844)
  line L750 (8.9656, 7.844) -> (9.1437, 7.8641)
  line L751 (9.1437, 7.8641) -> (9.3217, 7.844)
  line L752 (6.7817, 7.844) -> (6.9508, 7.7849)
  line L753 (6.9508, 7.7849) -> (7.1025, 7.6896)
  line L754 (7.1025, 7.6896) -> (7.2291, 7.5629)
  line L755 (7.2291, 7.5629) -> (7.3244, 7.4112)
  line L756 (7.3244, 7.4112) -> (7.3836, 7.2421)
  line L757 (7.3836, 7.2421) -> (7.4037, 7.0641)
  line L758 (7.4037, 7.0641) -> (7.3836, 6.8861)
  line L759 (7.3836, 6.8861) -> (7.3244, 6.717)
  line L760 (7.3244, 6.717) -> (7.2291, 6.5653)
  line L761 (7.2291, 6.5653) -> (7.1025, 6.4386)
  line L762 (7.1025, 6.4386) -> (6.9508, 6.3433)
  line L763 (6.9508, 6.3433) -> (6.7817, 6.2842)
  line L764 (6.7817, 6.2842) -> (6.6037, 6.2641)
  line L765 (6.6037, 6.2641) -> (6.4256, 6.2842)
  line L766 (6.4256, 6.2842) -> (6.2566, 6.3433)
  line L767 (6.2566, 6.3433) -> (6.1049, 6.4386)
  line L768 (6.1049, 6.4386) -> (5.9782, 6.5653)
  line L769 (5.9782, 6.5653) -> (5.8829, 6.717)
  line L770 (5.8829, 6.717) -> (5.8237, 6.8861)
  line L771 (5.8237, 6.8861) -> (5.8037, 7.0641)
  line L772 (5.8037, 7.0641) -> (5.8237, 7.2421)
  line L773 (5.8237, 7.2421) -> (5.8829, 7.4112)
  line L774 (5.8829, 7.4112) -> (5.9782, 7.5629)
  line L775 (5.9782, 7.5629) -> (6.1049, 7.6896)
  line L776 (6.1049, 7.6896) -> (6.2566, 7.7849)
  line L777 (6.2566, 7.7849) -> (6.4256, 7.844)
  line L778 (6.4256, 7.844) -> (6.6037, 7.8641)
  line L779 (6.6037, 7.8641) -> (6.7817, 7.844)
  line L780 (4.0637, 7.8641) -> (4.2417, 7.844)
  line L781 (4.2417, 7.844) -> (4.4108, 7.7849)
  line L782 (4.4108, 7.7849) -> (4.5625, 7.6896)
  line L783 (4.5625, 7.6896) -> (4.6891, 7.5629)
  line L784 (4.6891, 7.5629) -> (4.7844, 7.4112)
  line L785 (4.7844, 7.4112) -> (4.8436, 7.2421)
  line L786 (4.8436, 7.2421) -> (4.8637, 7.0641)
  line L787 (4.8637, 7.0641) -> (4.8436, 6.8861)
  line L788 (4.8436, 6.8861) -> (4.7844, 6.717)
  line L789 (4.7844, 6.717) -> (4.6891, 6.5653)
  line L790 (4.6891, 6.5653) -> (4.5625, 6.4386)
  line L791 (4.5625, 6.4386) -> (4.4108, 6.3433)
  line L792 (4.4108, 6.3433) -> (4.2417, 6.2842)
  line L793 (4.2417, 6.2842) -> (4.0637, 6.2641)
  line L794 (4.0637, 6.2641) -> (3.8856, 6.2842)
  line L795 (3.8856, 6.2842) -> (3.7166, 6.3433)
  line L796 (3.7166, 6.3433) -> (3.5649, 6.4386)
  line L797 (3.5649, 6.4386) -> (3.4382, 6.5653)
  line L798 (3.4382, 6.5653) -> (3.3429, 6.717)
  line L799 (3.3429, 6.717) -> (3.2837, 6.8861)
  line L800 (3.2837, 6.8861) -> (3.2637, 7.0641)
  line L801 (3.2637, 7.0641) -> (3.2837, 7.2421)
  line L802 (3.2837, 7.2421) -> (3.3429, 7.4112)
  line L803 (3.3429, 7.4112) -> (3.4382, 7.5629)
  line L804 (3.4382, 7.5629) -> (3.5649, 7.6896)
  line L805 (3.5649, 7.6896) -> (3.7166, 7.7849)
  line L806 (3.7166, 7.7849) -> (3.8856, 7.844)
  line L807 (3.8856, 7.844) -> (4.0637, 7.8641)
  line L808 (37.2617, 23.084) -> (37.4308, 23.0249)
  line L809 (37.4308, 23.0249) -> (37.5825, 22.9296)
  line L810 (37.5825, 22.9296) -> (37.7091, 22.8029)
  line L811 (37.7091, 22.8029) -> (37.8044, 22.6512)
  line L812 (37.8044, 22.6512) -> (37.8636, 22.4821)
  line L813 (37.8636, 22.4821) -> (37.8837, 22.3041)
  line L814 (37.8837, 22.3041) -> (37.8636, 22.1261)
  line L815 (37.8636, 22.1261) -> (37.8044, 21.957)
  line L816 (37.8044, 21.957) -> (37.7091, 21.8053)
  line L817 (37.7091, 21.8053) -> (37.5837, 21.6798)
  line L818 (37.5837, 21.6798) -> (37.5837, 16.3234)
  line L819 (37.5837, 16.3234) -> (39.7771, 14.13)
  line L820 (39.7771, 14.13) -> (42.4257, 14.13)
  line L821 (42.4257, 14.13) -> (42.5512, 14.2555)
  line L822 (42.5512, 14.2555) -> (42.7029, 14.3508)
  line L823 (42.7029, 14.3508) -> (42.872, 14.4099)
  line L824 (42.872, 14.4099) -> (43.05, 14.43)
  line L825 (43.05, 14.43) -> (43.228, 14.4099)
  line L826 (43.228, 14.4099) -> (43.3971, 14.3508)
  line L827 (43.3971, 14.3508) -> (43.5488, 14.2555)
  line L828 (43.5488, 14.2555) -> (43.6755, 14.1288)
  line L829 (43.6755, 14.1288) -> (43.7708, 13.9771)
  line L830 (43.7708, 13.9771) -> (43.8299, 13.808)
  line L831 (43.8299, 13.808) -> (43.85, 13.63)
  line L832 (43.85, 13.63) -> (43.8299, 13.452)
  line L833 (43.8299, 13.452) -> (43.7708, 13.2829)
  line L834 (43.7708, 13.2829) -> (43.6755, 13.1312)
  line L835 (43.6755, 13.1312) -> (43.5488, 13.0045)
  line L836 (43.5488, 13.0045) -> (43.3971, 12.9092)
  line L837 (43.3971, 12.9092) -> (43.228, 12.8501)
  line L838 (43.228, 12.8501) -> (43.05, 12.83)
  line L839 (43.05, 12.83) -> (42.872, 12.8501)
  line L840 (42.872, 12.8501) -> (42.7029, 12.9092)
  line L841 (42.7029, 12.9092) -> (42.5512, 13.0045)
  line L842 (42.5512, 13.0045) -> (42.4257, 13.13)
  line L843 (42.4257, 13.13) -> (39.57, 13.13)
  line L844 (39.57, 13.13) -> (39.5171, 13.1376)
  line L845 (39.5171, 13.1376) -> (39.4637, 13.1414)
  line L846 (39.4637, 13.1414) -> (39.4469, 13.1477)
  line L847 (39.4469, 13.1477) -> (39.4291, 13.1503)
  line L848 (39.4291, 13.1503) -> (39.3805, 13.1725)
  line L849 (39.3805, 13.1725) -> (39.3304, 13.1912)
  line L850 (39.3304, 13.1912) -> (39.316, 13.2019)
  line L851 (39.316, 13.2019) -> (39.2997, 13.2094)
  line L852 (39.2997, 13.2094) -> (39.2593, 13.2444)
  line L853 (39.2593, 13.2444) -> (39.2164, 13.2764)
  line L854 (39.2164, 13.2764) -> (36.6964, 15.7964)
  line L855 (36.6964, 15.7964) -> (36.675, 15.8251)
  line L856 (36.675, 15.8251) -> (36.6497, 15.8504)
  line L857 (36.6497, 15.8504) -> (36.6326, 15.8818)
  line L858 (36.6326, 15.8818) -> (36.6112, 15.9104)
  line L859 (36.6112, 15.9104) -> (36.5987, 15.9439)
  line L860 (36.5987, 15.9439) -> (36.5815, 15.9753)
  line L861 (36.5815, 15.9753) -> (36.5739, 16.0102)
  line L862 (36.5739, 16.0102) -> (36.5614, 16.0437)
  line L863 (36.5614, 16.0437) -> (36.5589, 16.0794)
  line L864 (36.5589, 16.0794) -> (36.5513, 16.1143)
  line L865 (36.5513, 16.1143) -> (36.5538, 16.15)
  line L866 (36.5538, 16.15) -> (36.5513, 16.1857)
  line L867 (36.5513, 16.1857) -> (36.5589, 16.2206)
  line L868 (36.5589, 16.2206) -> (36.5614, 16.2563)
  line L869 (36.5614, 16.2563) -> (36.5739, 16.2898)
  line L870 (36.5739, 16.2898) -> (36.5815, 16.3247)
  line L871 (36.5815, 16.3247) -> (36.5837, 16.3286)
  line L872 (36.5837, 16.3286) -> (36.5837, 21.6798)
  line L873 (36.5837, 21.6798) -> (36.4582, 21.8053)
  line L874 (36.4582, 21.8053) -> (36.3629, 21.957)
  line L875 (36.3629, 21.957) -> (36.3037, 22.1261)
  line L876 (36.3037, 22.1261) -> (36.2837, 22.3041)
  line L877 (36.2837, 22.3041) -> (36.3037, 22.4821)
  line L878 (36.3037, 22.4821) -> (36.3629, 22.6512)
  line L879 (36.3629, 22.6512) -> (36.4582, 22.8029)
  line L880 (36.4582, 22.8029) -> (36.5849, 22.9296)
  line L881 (36.5849, 22.9296) -> (36.7366, 23.0249)
  line L882 (36.7366, 23.0249) -> (36.9056, 23.084)
  line L883 (36.9056, 23.084) -> (37.0837, 23.1041)
  line L884 (37.0837, 23.1041) -> (37.2617, 23.084)
  line L885 (40.4237, 21.5041) -> (40.1237, 21.5041)
  line L886 (40.1237, 21.5041) -> (40.1237, 17.6834)
  line L887 (40.1237, 17.6834) -> (41.1371, 16.67)
  line L888 (41.1371, 16.67) -> (42.4257, 16.67)
  line L889 (42.4257, 16.67) -> (42.5512, 16.7955)
  line L890 (42.5512, 16.7955) -> (42.7029, 16.8908)
  line L891 (42.7029, 16.8908) -> (42.872, 16.9499)
  line L892 (42.872, 16.9499) -> (43.05, 16.97)
  line L893 (43.05, 16.97) -> (43.228, 16.9499)
  line L894 (43.228, 16.9499) -> (43.3971, 16.8908)
  line L895 (43.3971, 16.8908) -> (43.5488, 16.7955)
  line L896 (43.5488, 16.7955) -> (43.6755, 16.6688)
  line L897 (43.6755, 16.6688) -> (43.7708, 16.5171)
  line L898 (43.7708, 16.5171) -> (43.8299, 16.348)
  line L899 (43.8299, 16.348) -> (43.85, 16.17)
  line L900 (43.85, 16.17) -> (43.8299, 15.992)
  line L901 (43.8299, 15.992) -> (43.7708, 15.8229)
  line L902 (43.7708, 15.8229) -> (43.6755, 15.6712)
  line L903 (43.6755, 15.6712) -> (43.5488, 15.5445)
  line L904 (43.5488, 15.5445) -> (43.3971, 15.4492)
  line L905 (43.3971, 15.4492) -> (43.228, 15.3901)
  line L906 (43.228, 15.3901) -> (43.05, 15.37)
  line L907 (43.05, 15.37) -> (42.872, 15.3901)
  line L908 (42.872, 15.3901) -> (42.7029, 15.4492)
  line L909 (42.7029, 15.4492) -> (42.5512, 15.5445)
  line L910 (42.5512, 15.5445) -> (42.4257, 15.67)
  line L911 (42.4257, 15.67) -> (40.93, 15.67)
  line L912 (40.93, 15.67) -> (40.8771, 15.6776)
  line L913 (40.8771, 15.6776) -> (40.8237, 15.6814)
  line L914 (40.8237, 15.6814) -> (40.8069, 15.6877)
  line L915 (40.8069, 15.6877) -> (40.7891, 15.6903)
  line L916 (40.7891, 15.6903) -> (40.7405, 15.7125)
  line L917 (40.7405, 15.7125) -> (40.6904, 15.7312)
  line L918 (40.6904, 15.7312) -> (40.676, 15.7419)
  line L919 (40.676, 15.7419) -> (40.6597, 15.7494)
  line L920 (40.6597, 15.7494) -> (40.6193, 15.7844)
  line L921 (40.6193, 15.7844) -> (40.5764, 15.8164)
  line L922 (40.5764, 15.8164) -> (39.2701, 17.1228)
  line L923 (39.2701, 17.1228) -> (39.2381, 17.1656)
  line L924 (39.2381, 17.1656) -> (39.203, 17.206)
  line L925 (39.203, 17.206) -> (39.1956, 17.2223)
  line L926 (39.1956, 17.2223) -> (39.1848, 17.2367)
  line L927 (39.1848, 17.2367) -> (39.1661, 17.2868)
  line L928 (39.1661, 17.2868) -> (39.1439, 17.3355)
  line L929 (39.1439, 17.3355) -> (39.1414, 17.3532)
  line L930 (39.1414, 17.3532) -> (39.1351, 17.3701)
  line L931 (39.1351, 17.3701) -> (39.1313, 17.4234)
  line L932 (39.1313, 17.4234) -> (39.1237, 17.4763)
  line L933 (39.1237, 17.4763) -> (39.1237, 21.5041)
  line L934 (39.1237, 21.5041) -> (38.8237, 21.5041)
  line L935 (38.8237, 21.5041) -> (38.8237, 23.1041)
  line L936 (38.8237, 23.1041) -> (40.4237, 23.1041)
  line L937 (40.4237, 23.1041) -> (40.4237, 21.5041)
  line L938 (43.228, 19.4899) -> (43.3971, 19.4308)
  line L939 (43.3971, 19.4308) -> (43.5488, 19.3355)
  line L940 (43.5488, 19.3355) -> (43.6755, 19.2088)
  line L941 (43.6755, 19.2088) -> (43.7708, 19.0571)
  line L942 (43.7708, 19.0571) -> (43.8299, 18.888)
  line L943 (43.8299, 18.888) -> (43.85, 18.71)
  line L944 (43.85, 18.71) -> (43.8299, 18.532)
  line L945 (43.8299, 18.532) -> (43.7708, 18.3629)
  line L946 (43.7708, 18.3629) -> (43.6755, 18.2112)
  line L947 (43.6755, 18.2112) -> (43.5488, 18.0845)
  line L948 (43.5488, 18.0845) -> (43.3971, 17.9892)
  line L949 (43.3971, 17.9892) -> (43.228, 17.9301)
  line L950 (43.228, 17.9301) -> (43.05, 17.91)
  line L951 (43.05, 17.91) -> (42.872, 17.9301)
  line L952 (42.872, 17.9301) -> (42.7029, 17.9892)
  line L953 (42.7029, 17.9892) -> (42.5512, 18.0845)
  line L954 (42.5512, 18.0845) -> (42.4245, 18.2112)
  line L955 (42.4245, 18.2112) -> (42.3292, 18.3629)
  line L956 (42.3292, 18.3629) -> (42.2701, 18.532)
  line L957 (42.2701, 18.532) -> (42.25, 18.71)
  line L958 (42.25, 18.71) -> (42.2701, 18.888)
  line L959 (42.2701, 18.888) -> (42.3292, 19.0571)
  line L960 (42.3292, 19.0571) -> (42.4245, 19.2088)
  line L961 (42.4245, 19.2088) -> (42.5512, 19.3355)
  line L962 (42.5512, 19.3355) -> (42.7029, 19.4308)
  line L963 (42.7029, 19.4308) -> (42.872, 19.4899)
  line L964 (42.872, 19.4899) -> (43.05, 19.51)
  line L965 (43.05, 19.51) -> (43.228, 19.4899)
  line L966 (34.7217, 23.084) -> (34.8908, 23.0249)
  line L967 (34.8908, 23.0249) -> (35.0425, 22.9296)
  line L968 (35.0425, 22.9296) -> (35.1691, 22.8029)
  line L969 (35.1691, 22.8029) -> (35.2644, 22.6512)
  line L970 (35.2644, 22.6512) -> (35.3236, 22.4821)
  line L971 (35.3236, 22.4821) -> (35.3437, 22.3041)
  line L972 (35.3437, 22.3041) -> (35.3236, 22.1261)
  line L973 (35.3236, 22.1261) -> (35.2644, 21.957)
  line L974 (35.2644, 21.957) -> (35.1691, 21.8053)
  line L975 (35.1691, 21.8053) -> (35.0425, 21.6786)
  line L976 (35.0425, 21.6786) -> (34.8908, 21.5833)
  line L977 (34.8908, 21.5833) -> (34.7217, 21.5241)
  line L978 (34.7217, 21.5241) -> (34.5437, 21.5041)
  line L979 (34.5437, 21.5041) -> (34.3656, 21.5241)
  line L980 (34.3656, 21.5241) -> (34.1966, 21.5833)
  line L981 (34.1966, 21.5833) -> (34.0449, 21.6786)
  line L982 (34.0449, 21.6786) -> (33.9182, 21.8053)